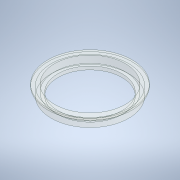
# Autodesk Inventor part: внешнее кольцо подшипника
Saved by Autodesk Inventor 2020.1 (Build 241239000, 239)
## iProperties
Created: 2022-04-01
Part Number: внешнее кольцо подшипника
Material: Стекло
Document SubType Name: Modeling
Designer: User
Density: 2.18 g/cm^3
Appearance: Бесцветный
Author: User
Autodesk Inventor part; units mm, degrees
ref_plane "YZ Plane" through (0, 0, 0) normal (1, 0, 0) x (0, 1, 0)
ref_plane "XZ Plane" through (0, 0, 0) normal (0, 1, 0) x (-1, 0, 0)
ref_plane "XY Plane" through (0, 0, 0) normal (0, 0, 1) x (1, 0, 0)
sketch "Эскиз1" plane through (0, 0, 0) normal (0, 1, 0) x (-1, 0, 0)
  circle A0 centre (0, 0) radius 46.5
  circle A1 centre (0, 0) radius 38.5
  point P0 (0, 38.5)
  point P1 (0, 46.5)
  dimension "d0" = 93
  dimension "d3" = 8
  constraints: 2 coincident, 2 vertical alignment, 4 other
  measures "d3" distance of point (0, 46.5) point (0, 38.5)
extrude "Выдавливание1" add sketch "Эскиз1" along normal blind 4
sketch "Эскиз2" plane through (0, 4, 0) normal (0, 1, 0) x (1, 0, 0)
  circle A0 centre (0, 0) radius 46.5
  circle A1 centre (0, 0) radius 42.5
  circle A2 centre (0, 0) radius 46.5 projected
  point P0 (0, -42.5)
  point P1 (0, -46.5)
  point P2 (0, -46.5)
  dimension "d4" = 4
  dimension "d5" = 0
  constraints: 3 vertical alignment, 2 coincident, 5 other
  measures "d4" distance of point (0, -42.5) point (0, -46.5)
  measures "d5" distance of point (0, -46.5) point (0, -46.5)
extrude "Выдавливание2" add sketch "Эскиз2" along normal blind 8.5
sketch "Эскиз3" plane through (0, 12.5, 0) normal (0, 1, 0) x (1, 0, 0)
  circle A0 centre (0, 0) radius 46.5
  circle A1 centre (0, 0) radius 50.5
  circle A2 centre (0, 0) radius 46.5 projected
  point P0 (-46.5, 0)
  point P1 (-50.5, 0)
  dimension "d8" = 93
  dimension "d9" = 4
  constraints: 2 coincident, 2 horizontal alignment, 1 centre point, 3 other
  measures "d8" diameter of A0
  measures "d9" distance of point (-50.5, 0) point (-46.5, 0)
extrude "Выдавливание3" add sketch "Эскиз3" against normal blind 2
